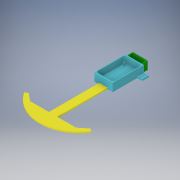
# Autodesk Inventor part: Body
Saved by Autodesk Inventor 2019.3 (Build 233278000, 278)
## iProperties
Created: 2019-03-27
Part Number: Body
Material: Generic
Document SubType Name: Modeling
Designer: oskar
Density: 1 g/cm^3
Appearance: Default
Author: oskar
Autodesk Inventor part; units mm, degrees
ref_plane "YZ Plane" through (0, 0, 0) normal (1, 0, 0) x (0, 1, 0)
ref_plane "XZ Plane" through (0, 0, 0) normal (0, 1, 0) x (-1, 0, 0)
ref_plane "XY Plane" through (0, 0, 0) normal (0, 0, 1) x (1, 0, 0)
sketch "Sketch1" plane through (0, 0, 0) normal (0, 1, 0) x (-1, 0, 0)
  line L0 (-21.69, 43) -> (21.69, 43)
  line L1 (25.5, 39.19) -> (25.5, -39.19)
  line L2 (21.69, -43) -> (-21.69, -43)
  line L3 (-25.5, -39.19) -> (-25.5, 39.19)
  line L4 (-25.5, 43) -> (25.5, -43) construction
  line L5 (25.5, 43) -> (-25.5, -43) construction
  line L6 (-25.5, 39.19) -> (-21.69, 43)
  line L7 (21.69, 43) -> (25.5, 39.19)
  line L8 (21.69, -43) -> (25.5, -39.19)
  line L9 (-25.5, -39.19) -> (-21.69, -43)
  line L10 (-27.5, 46.3725) -> (27.5, 46.3725)
  line L11 (27.5, 46.3725) -> (27.5, -46.3725)
  line L12 (27.5, -46.3725) -> (-27.5, -46.3725)
  line L13 (-27.5, -46.3725) -> (-27.5, 46.3725)
  line L14 (-27.5, 46.3725) -> (27.5, -46.3725) construction
  line L15 (27.5, 46.3725) -> (-27.5, -46.3725) construction
  point P0 (0, 0)
  dimension "d0" = 86
  dimension "d1" = 51
  dimension "d2" = 3.81
  dimension "d3" = 3.81
  dimension "d4" = 3.81
  dimension "d5" = 3.81
  dimension "d6" = 3.81
  dimension "d7" = 3.81
  dimension "d8" = 3.81
  dimension "d9" = 3.81
  dimension "d10" = 2
  constraints: 32 end point, 8 point on line, 4 midpoint, 4 parallel, 2 horizontal, 2 perpendicular, 1 collinear
  measures "d0" distance of L5.start L4.end
  measures "d1" distance of L4.end L5.end
  measures "d2" distance of L3.end L4.start
  measures "d3" distance of L0.start L4.start
  measures "d4" distance of L0.end L5.start
  measures "d5" distance of L1.start L5.start
  measures "d6" distance of L2.start L4.end
  measures "d7" distance of L1.end L4.end
  measures "d8" distance of L3.start L5.end
  measures "d9" distance of L2.end L5.end
  measures "d10" distance from line of L11 L1.end
extrude "Extrusion1" add sketch "Sketch1" along normal blind 20
sketch "Sketch2" plane through (0, 0, 0) normal (0, 1, 0) x (-1, 0, 0)
  circle A0 centre (20, 35) radius 2.5
  line L0 (0, -52.5) -> (0, 52.5) projected
  line L1 (31.5, 0) -> (-31.5, 0) projected
  circle A1 centre (20, 35) radius 1
  circle A2 centre (20, -35) radius 2.5
  circle A3 centre (20, -35) radius 1
  circle A4 centre (-20, 35) radius 2.5
  circle A5 centre (-20, 35) radius 1
  circle A6 centre (-20, -35) radius 2.5
  circle A7 centre (-20, -35) radius 1
  point P0 (0, 0)
  dimension "d13" = 5
  dimension "d14" = 2
  dimension "d15" = 40
  dimension "d16" = 70
  constraints: 8 centre point, 6 symmetric about line, 4 coincident, 6 other
  measures "d13" diameter of A0
  measures "d14" diameter of A1
  measures "d15" distance of A6.centre A2.centre
  measures "d16" distance of A4.centre A6.centre
extrude "Extrusion2" add sketch "Sketch2" along normal blind 8 contours A0 | A1 | A2 | A3 | A4 | A5 | A6 | A7
extrude "Extrusion3" add sketch "Sketch2" along normal blind 10 contours A1 | A3 | A5 | A7
sketch "Sketch3" plane through (0, 0, 0) normal (0, -1, 0) x (1, 0, 0)
  line L0 (-21.69, 43) -> (21.69, 43) projected
  line L1 (21.69, 43) -> (25.5, 39.19) projected
  line L2 (25.5, 39.19) -> (25.5, -39.19) projected
  line L3 (25.5, -39.19) -> (21.69, -43) projected
  line L4 (21.69, -43) -> (-21.69, -43) projected
  line L5 (-21.69, -43) -> (-25.5, -39.19) projected
  line L6 (-25.5, -39.19) -> (-25.5, 39.19) projected
  line L7 (-25.5, 39.19) -> (-21.69, 43) projected
  line L8 (27.5, 46.3725) -> (-27.5, 46.3725) projected
  line L9 (-27.5, 46.3725) -> (-27.5, -46.3725) projected
  line L10 (-27.5, -46.3725) -> (27.5, -46.3725) projected
  line L11 (27.5, -46.3725) -> (27.5, 46.3725) projected
  point P0 (0, 0)
extrude "Extrusion4" add sketch "Sketch3" along normal blind 4 contours L0 L1 L2 L3 L4 L5 L6 L7 | L11 L10 L9 L8
sketch "Sketch4" plane through (0, 0, 0) normal (0, 1, 0) x (-1, 0, 0)
  line L0 (0, -39.2745) -> (0, 235.6471) projected
  line L1 (-12.5, 196.3725) -> (12.5, 196.3725)
  line L2 (12.5, 196.3725) -> (12.5, 46.3725)
  line L3 (12.5, 46.3725) -> (-12.5, 46.3725)
  line L4 (-12.5, 46.3725) -> (-12.5, 196.3725)
  line L5 (-12.5, 196.3725) -> (12.5, 46.3725) construction
  line L6 (12.5, 196.3725) -> (-12.5, 46.3725) construction
  line L7 (27.5, 46.3725) -> (-27.5, 46.3725) projected
  point P0 (0, 0)
  point P1 (0, 121.3725)
  dimension "d23" = 25
  dimension "d24" = 150
  constraints: 12 end point, 2 midpoint, 2 parallel, 1 collinear, 1 horizontal, 1 perpendicular, 1 point on line
  measures "d23" distance between parallel lines of L4 L2
  measures "d24" distance between parallel lines of L1 L3
extrude "Extrusion5" add sketch "Sketch4" against normal blind 4 separate body
sketch "Sketch5" plane through (0, -4, 0) normal (0, -1, 0) x (1, 0, 0)
  line L0 (0, -102.9216) -> (0, 292.9216) projected
  arc A0 (100, 182.705) -> (-100, 182.705) centre (0, 116.3725) ccw
  line L1 (100, 182.705) -> (91.6667, 177.1773)
  line L2 (91.6667, 177.1773) -> (68.6114, 196.3725)
  line L3 (68.6114, 196.3725) -> (0, 196.3725)
  line L4 (-100, 182.705) -> (-91.6667, 177.1773)
  line L5 (-91.6667, 177.1773) -> (-68.6114, 196.3725)
  line L6 (-68.6114, 196.3725) -> (0, 196.3725)
  line L7 (12.5, 196.3725) -> (-12.5, 196.3725) projected
  point P0 (0, 0)
  dimension "d29" = 120
  dimension "d31" = 100
  dimension "d32" = 100
  dimension "d33" = 10
  dimension "d34" = 80
  dimension "d35" = 30
  constraints: 12 end point, 2 line through centre, 2 point on circle, 2 point on line, 2 symmetric about line, 1 centre point, 1 collinear, 1 perpendicular
  measures "d29" radius of A0
  measures "d31" distance from line of L1.start L0
  measures "d32" distance from line of L0 L4.start
  measures "d33" distance of L1.start L1.end
  measures "d34" distance from line of L3 A0.centre
  measures "d35" distance of L1.end L2.end
extrude "Extrusion6" add sketch "Sketch5" against normal blind 4 bodies 2
sketch "Sketch6" plane through (0, 0, 0) normal (0, 1, 0) x (-1, 0, 0)
  line L0 (-20, -46.3725) -> (20, -46.3725)
  line L1 (20, -46.3725) -> (20, -61.3725)
  line L2 (20, -61.3725) -> (-20, -61.3725)
  line L3 (-20, -61.3725) -> (-20, -46.3725)
  line L4 (-20, -46.3725) -> (20, -61.3725) construction
  line L5 (20, -46.3725) -> (-20, -61.3725) construction
  line L6 (-27.5, -46.3725) -> (27.5, -46.3725) projected
  line L7 (-22, -63.3725) -> (22, -63.3725)
  line L8 (22, -63.3725) -> (22, -46.3725)
  line L9 (22, -46.3725) -> (-22, -46.3725)
  line L10 (-22, -46.3725) -> (-22, -63.3725)
  line L11 (-22, -63.3725) -> (22, -46.3725) construction
  line L12 (22, -63.3725) -> (-22, -46.3725) construction
  line L13 (0, -76.0471) -> (0, 12.6745) projected
  point P0 (0, 0)
  point P1 (0, -53.8725)
  point P2 (0, -54.8725)
  point P3 (0, -54.8725)
  point P4 (0, -53.8725)
  dimension "d38" = 40
  dimension "d39" = 15
  dimension "d40" = 2
  dimension "d41" = 2
  constraints: 24 end point, 6 midpoint, 4 parallel, 3 point on line, 2 horizontal, 2 perpendicular, 1 collinear
  measures "d38" distance of L1.end L2.end
  measures "d39" distance of L0.end L1.end
  measures "d40" distance between parallel lines of L8 L1
  measures "d41" distance between parallel lines of L7 L2
extrude "Extrusion7" add sketch "Sketch6" along normal blind 20 separate body contours L3 L2 L13 L7 L10 L6 | L6 L8 L7 L13 L2 L1
extrude "Extrusion8" add sketch "Sketch6" against normal blind 4 bodies 3
sketch "Sketch7" plane through (0, 0, 0) normal (0, 1, 0) x (-1, 0, 0)
  line L0 (-27.5, -26.3725) -> (-42.5, -26.3725)
  line L1 (-42.5, -26.3725) -> (-42.5, -46.3725)
  line L2 (-42.5, -46.3725) -> (-27.5, -46.3725)
  line L3 (-27.5, -46.3725) -> (-27.5, -26.3725)
  line L4 (-27.5, -26.3725) -> (-42.5, -46.3725) construction
  line L5 (-42.5, -26.3725) -> (-27.5, -46.3725) construction
  line L6 (-27.5, 46.3725) -> (-27.5, -46.3725) projected
  line L7 (-27.5, -46.3725) -> (27.5, -46.3725) projected
  line L8 (0, -123.3216) -> (0, 296.3216) projected
  line L9 (27.5, -26.3725) -> (42.5, -26.3725)
  line L10 (42.5, -26.3725) -> (42.5, -46.3725)
  line L11 (42.5, -46.3725) -> (27.5, -46.3725)
  line L12 (27.5, -46.3725) -> (27.5, -26.3725)
  point P0 (0, 0)
  point P1 (-35, -36.3725)
  dimension "d46" = 20
  dimension "d47" = 15
  constraints: 20 end point, 4 symmetric about line, 2 collinear, 2 midpoint, 2 parallel, 1 horizontal, 1 perpendicular
  measures "d46" distance between parallel lines of L2 L0
  measures "d47" distance between parallel lines of L1 L3
extrude "Extrusion9" add sketch "Sketch7" against normal blind 4 bodies 1
sketch "Sketch8" plane through (0, 0, 0) normal (0, 1, 0) x (1, 0, 0)
  line L0 (-55.7062, 36.3725) -> (-34.5441, 36.3725) construction
  line L1 (-42.5, 46.3725) -> (-27.5, 46.3725) projected
  line L2 (-42.5, 26.3725) -> (-42.5, 46.3725) projected
  line L3 (0, 123.3216) -> (0, -296.3216) projected
  point P0 (0, 0)
  point P1 (-37.5, 31.3725)
  point P2 (-37.5, 41.3725)
  point P3 (37.5, 31.3725)
  point P4 (37.5, 41.3725)
  dimension "d50" = 10
  dimension "d51" = 10
  dimension "d52" = 5
  constraints: 3 symmetric about line, 2 end point, 1 horizontal
  measures "d50" distance between parallel lines of L0 L1
  measures "d51" distance of point (-37.5, 41.373) point (-37.5, 31.373)
  measures "d52" distance from line of L2 point (-37.5, 41.373)
hole "Hole1" at (-37.5, 0, -31.3725) at (-37.5, 0, -41.3725) at (37.5, 0, -31.3725) at (37.5, 0, -41.3725) direction (0, -1, 0) diameter 2.5 end through all bodies 1
equation "\"d2\" = Chamfer_PCB"
equation "\"d3\" = d2"
equation "\"d4\" = Chamfer_PCB"
equation "\"d5\" = d4"
equation "\"d6\" = Chamfer_PCB"
equation "\"d7\" = d6"
equation "\"d8\" = Chamfer_PCB"
equation "\"d9\" = d8"
equation "\"d11\" = 2 * HU_PCB"
equation "\"d15\" = DIH_PCB"
equation "\"d16\" = DOH_PCB"
equation "\"d19\" = HU_PCB"
equation "\"d21\" = H_Wall"
equation "\"d23\" = 0.5 * W_PCB"
equation "\"d24\" = L_PCBToSensor"
equation "\"d25\" = H_Wall"
equation "\"d31\" = 0.5 * W_MaxWidth"
equation "\"d32\" = d31"
equation "\"d36\" = H_Wall"
equation "\"d38\" = L_LiPo_245mAh"
equation "\"d39\" = H_LiPo_245mAh"
equation "\"d40\" = 0.5 * H_Wall"
equation "\"d41\" = d40"
equation "\"d42\" = W_LiPo_245mAh"
equation "\"d44\" = H_Wall"
equation "\"d46\" = 2 * DSH_Motor"
equation "\"d48\" = H_Wall"
equation "\"d50\" = DSH_Motor"
equation "\"d51\" = DSH_Motor"
equation "\"d52\" = 0.5 * DSH_Motor"
equation "\"HU_PCB\" = 10"
equation "\"L_PCB\" = 85"
equation "\"DIH_PCB\" = 40"
equation "\"DOH_PCB\" = 70"
equation "\"Chamfer_PCB\" = 3.81"
equation "\"L_PCBToSensor\" = 150"
equation "\"H_Wall\" = 4"
equation "\"W_LiPo_245mAh\" = 20"
equation "\"H_LiPo_245mAh\" = 15"
equation "\"L_LiPo_245mAh\" = 40"
equation "\"DSH_Motor\" = 10"
equation "\"W_PCB\" = 50"
equation "\"W_MaxWidth\" = 200"
body "Solid1"
body "Solid2"
body "Solid3"
